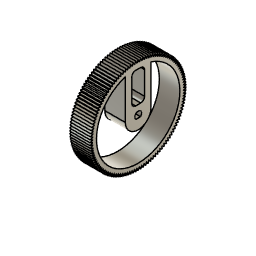
Whell Medium (Autodesk Fusion 360 design; units mm, degrees)
Autodesk Fusion 360 part; units mm, degrees
sketch "Sketch1" plane through (34, 0, 0) normal (-1, 0, 0) x (0, -1, 0)
  arc A0 (1.8888, -2) -> (-1.7388, -2) centre (0.075, 0) ccw
  line L0 (1.8888, -2) -> (-1.7388, -2)
  arc A1 (41.9734, -20.1687) -> (37.4682, -13) centre (37.4682, -18) ccw
  arc A2 (41.9734, 20.1687) -> (41.9734, -20.1687) centre (0.075, 0) ccw
  arc A3 (37.4682, 13) -> (41.9734, 20.1687) centre (37.4682, 18) ccw
  arc A4 (43.369, 3) -> (36.369, 10) centre (36.369, 3) ccw
  line L1 (43.369, 3) -> (43.369, -2.9712)
  arc A5 (36.369, -9.9712) -> (43.369, -2.9712) centre (36.369, -2.9712) ccw
  arc A6 (14.223, -2.9712) -> (21.223, -9.9712) centre (21.223, -2.9712) ccw
  line L2 (14.223, -2.9712) -> (14.223, 3)
  arc A7 (21.223, 10) -> (14.223, 3) centre (21.223, 3) ccw
  arc A8 (50.075, -0.0217) -> (50.075, 0.0217) centre (0.075, 0) ccw
  line L3 (50.075, 0.0217) -> (51.2929, 5.3832)
  line L4 (51.2929, 5.3832) -> (48.9869, 10.3743)
  arc A9 (48.9869, 10.3743) -> (48.9779, 10.4168) centre (0.075, 0) ccw
  line L5 (48.9779, 10.4168) -> (49.0544, 15.9144)
  line L6 (49.0544, 15.9144) -> (45.7611, 20.317)
  arc A10 (45.7611, 20.317) -> (45.7434, 20.3567) centre (0.075, 0) ccw
  line L7 (45.7434, 20.3567) -> (44.6753, 25.75)
  line L8 (44.6753, 25.75) -> (40.5386, 29.3717)
  arc A11 (40.5386, 29.3717) -> (40.5131, 29.4068) centre (0.075, 0) ccw
  line L9 (40.5131, 29.4068) -> (38.347, 34.4602)
  line L10 (38.347, 34.4602) -> (33.5477, 37.1427)
  arc A12 (33.5477, 37.1427) -> (33.5154, 37.1718) centre (0.075, 0) ccw
  line L11 (33.5154, 37.1718) -> (30.3459, 41.6644)
  line L12 (30.3459, 41.6644) -> (25.0938, 43.2904)
  arc A13 (25.0938, 43.2904) -> (25.0562, 43.3121) centre (0.075, 0) ccw
  line L13 (25.0562, 43.3121) -> (21.0219, 47.0476)
  line L14 (21.0219, 47.0476) -> (15.5465, 47.5461)
  arc A14 (15.5465, 47.5461) -> (15.5052, 47.5595) centre (0.075, 0) ccw
  line L15 (15.5052, 47.5595) -> (10.7825, 50.3746)
  line L16 (10.7825, 50.3746) -> (5.323, 49.7238)
  arc A15 (5.323, 49.7238) -> (5.2798, 49.7284) centre (0.075, 0) ccw
  line L17 (5.2798, 49.7284) -> (0.075, 51.5)
  line L18 (0.075, 51.5) -> (-5.1298, 49.7284)
  arc A16 (-5.1298, 49.7284) -> (-5.173, 49.7238) centre (0.075, 0) ccw
  line L19 (-5.173, 49.7238) -> (-10.6325, 50.3746)
  line L20 (-10.6325, 50.3746) -> (-15.3552, 47.5595)
  arc A17 (-15.3552, 47.5595) -> (-15.3965, 47.5461) centre (0.075, 0) ccw
  line L21 (-15.3965, 47.5461) -> (-20.8719, 47.0476)
  line L22 (-20.8719, 47.0476) -> (-24.9062, 43.3121)
  arc A18 (-24.9062, 43.3121) -> (-24.9438, 43.2904) centre (0.075, 0) ccw
  line L23 (-24.9438, 43.2904) -> (-30.1959, 41.6644)
  line L24 (-30.1959, 41.6644) -> (-33.3654, 37.1718)
  arc A19 (-33.3654, 37.1718) -> (-33.3977, 37.1427) centre (0.075, 0) ccw
  line L25 (-33.3977, 37.1427) -> (-38.197, 34.4602)
  line L26 (-38.197, 34.4602) -> (-40.3631, 29.4068)
  arc A20 (-40.3631, 29.4068) -> (-40.3886, 29.3717) centre (0.075, 0) ccw
  line L27 (-40.3886, 29.3717) -> (-44.5253, 25.75)
  line L28 (-44.5253, 25.75) -> (-45.5934, 20.3567)
  arc A21 (-45.5934, 20.3567) -> (-45.6111, 20.317) centre (0.075, 0) ccw
  line L29 (-45.6111, 20.317) -> (-48.9044, 15.9144)
  line L30 (-48.9044, 15.9144) -> (-48.8279, 10.4168)
  arc A22 (-48.8279, 10.4168) -> (-48.8369, 10.3743) centre (0.075, 0) ccw
  line L31 (-48.8369, 10.3743) -> (-51.1429, 5.3832)
  line L32 (-51.1429, 5.3832) -> (-49.925, 0.0217)
  arc A23 (-49.925, 0.0217) -> (-49.925, -0.0217) centre (0.075, 0) ccw
  line L33 (-49.925, -0.0217) -> (-51.1429, -5.3832)
  line L34 (-51.1429, -5.3832) -> (-48.8369, -10.3743)
  arc A24 (-48.8369, -10.3743) -> (-48.8279, -10.4168) centre (0.075, 0) ccw
  line L35 (-48.8279, -10.4168) -> (-48.9044, -15.9144)
  line L36 (-48.9044, -15.9144) -> (-45.6111, -20.317)
  arc A25 (-45.6111, -20.317) -> (-45.5934, -20.3567) centre (0.075, 0) ccw
  line L37 (-45.5934, -20.3567) -> (-44.5253, -25.75)
  line L38 (-44.5253, -25.75) -> (-40.3886, -29.3717)
  arc A26 (-40.3886, -29.3717) -> (-40.3631, -29.4068) centre (0.075, 0) ccw
  line L39 (-40.3631, -29.4068) -> (-38.197, -34.4602)
  line L40 (-38.197, -34.4602) -> (-33.3977, -37.1427)
  arc A27 (-33.3977, -37.1427) -> (-33.3654, -37.1718) centre (0.075, 0) ccw
  line L41 (-33.3654, -37.1718) -> (-30.1959, -41.6644)
  line L42 (-30.1959, -41.6644) -> (-24.9438, -43.2904)
  arc A28 (-24.9438, -43.2904) -> (-24.9062, -43.3121) centre (0.075, 0) ccw
  line L43 (-24.9062, -43.3121) -> (-20.8719, -47.0476)
  line L44 (-20.8719, -47.0476) -> (-15.3965, -47.5461)
  arc A29 (-15.3965, -47.5461) -> (-15.3552, -47.5595) centre (0.075, 0) ccw
  line L45 (-15.3552, -47.5595) -> (-10.6325, -50.3746)
  line L46 (-10.6325, -50.3746) -> (-5.173, -49.7238)
  arc A30 (-5.173, -49.7238) -> (-5.1298, -49.7284) centre (0.075, 0) ccw
  line L47 (-5.1298, -49.7284) -> (0.075, -51.5)
  line L48 (0.075, -51.5) -> (5.2798, -49.7284)
  arc A31 (5.2798, -49.7284) -> (5.323, -49.7238) centre (0.075, 0) ccw
  line L49 (5.323, -49.7238) -> (10.7825, -50.3746)
  line L50 (10.7825, -50.3746) -> (15.5052, -47.5595)
  arc A32 (15.5052, -47.5595) -> (15.5465, -47.5461) centre (0.075, 0) ccw
  line L51 (15.5465, -47.5461) -> (21.0219, -47.0476)
  line L52 (21.0219, -47.0476) -> (25.0562, -43.3121)
  arc A33 (25.0562, -43.3121) -> (25.0938, -43.2904) centre (0.075, 0) ccw
  line L53 (25.0938, -43.2904) -> (30.3459, -41.6644)
  line L54 (30.3459, -41.6644) -> (33.5154, -37.1718)
  arc A34 (33.5154, -37.1718) -> (33.5477, -37.1427) centre (0.075, 0) ccw
  line L55 (33.5477, -37.1427) -> (38.347, -34.4602)
  line L56 (38.347, -34.4602) -> (40.5131, -29.4068)
  arc A35 (40.5131, -29.4068) -> (40.5386, -29.3717) centre (0.075, 0) ccw
  line L57 (40.5386, -29.3717) -> (44.6753, -25.75)
  line L58 (44.6753, -25.75) -> (45.7434, -20.3567)
  arc A36 (45.7434, -20.3567) -> (45.7611, -20.317) centre (0.075, 0) ccw
  line L59 (45.7611, -20.317) -> (49.0544, -15.9144)
  line L60 (49.0544, -15.9144) -> (48.9779, -10.4168)
  arc A37 (48.9779, -10.4168) -> (48.9869, -10.3743) centre (0.075, 0) ccw
  line L61 (48.9869, -10.3743) -> (51.2929, -5.3832)
  line L62 (51.2929, -5.3832) -> (50.075, -0.0217)
  arc A38 (1.8888, -2) -> (-1.7388, -2) centre (0.075, 0) ccw
  line L63 (1.8888, -2) -> (-1.7388, -2)
  circle A39 centre (0.075, 0) radius 37.5
  line L64 (0.075, 0) -> (0.075, 37.5) construction
  line L65 (0.075, 37.5) -> (-1.0186, 34.9829)
  line L66 (0.075, 37.5) -> (1.1677, 34.9829)
  line L67 (-1.8876, 37.4486) -> (-0.6647, 34.9922)
  line L68 (-1.8876, 37.4486) -> (-2.8479, 34.8777)
  line L69 (-3.8448, 37.2946) -> (-2.495, 34.9055)
  line L70 (-3.8448, 37.2946) -> (-4.6693, 34.677)
  line L71 (-5.7913, 37.0383) -> (-4.3183, 34.7232)
  line L72 (-5.7913, 37.0383) -> (-6.4776, 34.3811)
  line L73 (-7.7217, 36.6805) -> (-6.1296, 34.4457)
  line L74 (-7.7217, 36.6805) -> (-8.268, 33.9911)
  line L75 (-9.6307, 36.2222) -> (-7.9238, 34.0737)
  line L76 (-9.6307, 36.2222) -> (-10.0355, 33.5079)
  line L77 (-11.5131, 35.6646) -> (-9.6961, 33.6084)
  line L78 (-11.5131, 35.6646) -> (-11.7754, 32.9328)
  line L79 (-13.3638, 35.0093) -> (-11.4417, 33.051)
  line L80 (-13.3638, 35.0093) -> (-13.4827, 32.2675)
  line L81 (-15.1776, 34.258) -> (-13.1556, 32.4029)
  line L82 (-15.1776, 34.258) -> (-15.1529, 31.5137)
  line L83 (-16.9496, 33.4127) -> (-14.8333, 31.6661)
  line L84 (-16.9496, 33.4127) -> (-16.7813, 30.6735)
  line L85 (-18.675, 32.476) -> (-16.4702, 30.8425)
  line L86 (-18.675, 32.476) -> (-18.3635, 29.7493)
  line L87 (-20.349, 31.4501) -> (-18.0617, 29.9343)
  line L88 (-20.349, 31.4501) -> (-19.8952, 28.7435)
  line L89 (-21.9669, 30.3381) -> (-19.6035, 28.9441)
  line L90 (-21.9669, 30.3381) -> (-21.3722, 27.659)
  line L91 (-23.5245, 29.143) -> (-21.0913, 27.8745)
  line L92 (-23.5245, 29.143) -> (-22.7903, 26.4986)
  line L93 (-25.0174, 27.8679) -> (-22.5211, 26.7285)
  line L94 (-25.0174, 27.8679) -> (-24.1458, 25.2656)
  line L95 (-26.4415, 26.5165) -> (-23.889, 25.5093)
  line L96 (-26.4415, 26.5165) -> (-25.4349, 23.9634)
  line L97 (-27.7929, 25.0924) -> (-25.1912, 24.2202)
  line L98 (-27.7929, 25.0924) -> (-26.6541, 22.5955)
  line L99 (-29.068, 23.5995) -> (-26.4242, 22.8646)
  line L100 (-29.068, 23.5995) -> (-27.8, 21.1656)
  line L101 (-30.2631, 22.0419) -> (-27.5845, 21.4465)
  line L102 (-30.2631, 22.0419) -> (-28.8696, 19.6777)
  line L103 (-31.3751, 20.424) -> (-28.669, 19.9695)
  line L104 (-31.3751, 20.424) -> (-29.8597, 18.1359)
  line L105 (-32.401, 18.75) -> (-29.6748, 18.4378)
  line L106 (-32.401, 18.75) -> (-30.7679, 16.5444)
  line L107 (-33.3377, 17.0246) -> (-30.599, 16.8555)
  line L108 (-33.3377, 17.0246) -> (-31.5915, 14.9075)
  line L109 (-34.183, 15.2526) -> (-31.4391, 15.2271)
  line L110 (-34.183, 15.2526) -> (-32.3283, 13.2298)
  line L111 (-34.9343, 13.4388) -> (-32.1928, 13.5569)
  line L112 (-34.9343, 13.4388) -> (-32.9763, 11.5158)
  line L113 (-35.5896, 11.5881) -> (-32.8581, 11.8495)
  line L114 (-35.5896, 11.5881) -> (-33.5337, 9.7703)
  line L115 (-36.1472, 9.7057) -> (-33.4331, 10.1097)
  line L116 (-36.1472, 9.7057) -> (-33.9989, 7.9979)
  line L117 (-36.6055, 7.7967) -> (-33.9163, 8.3422)
  line L118 (-36.6055, 7.7967) -> (-34.3708, 6.2037)
  line L119 (-36.9633, 5.8663) -> (-34.3063, 6.5518)
  line L120 (-36.9633, 5.8663) -> (-34.6483, 4.3924)
  line L121 (-37.2196, 3.9198) -> (-34.6021, 4.7434)
  line L122 (-37.2196, 3.9198) -> (-34.8306, 2.5691)
  line L123 (-37.3736, 1.9626) -> (-34.8028, 2.922)
  line L124 (-37.3736, 1.9626) -> (-34.9172, 0.7388)
  line L125 (-37.425, 0) -> (-34.9079, 1.0927)
  line L126 (-37.425, 0) -> (-34.9079, -1.0936)
  line L127 (-37.3736, -1.9626) -> (-34.9172, -0.7397)
  line L128 (-37.3736, -1.9626) -> (-34.8027, -2.9229)
  line L129 (-37.2196, -3.9198) -> (-34.8305, -2.57)
  line L130 (-37.2196, -3.9198) -> (-34.602, -4.7443)
  line L131 (-36.9633, -5.8663) -> (-34.6482, -4.3933)
  line L132 (-36.9633, -5.8663) -> (-34.3061, -6.5526)
  line L133 (-36.6055, -7.7967) -> (-34.3707, -6.2046)
  line L134 (-36.6055, -7.7967) -> (-33.9161, -8.343)
  line L135 (-36.1472, -9.7057) -> (-33.9987, -7.9988)
  line L136 (-36.1472, -9.7057) -> (-33.4329, -10.1105)
  line L137 (-35.5896, -11.5881) -> (-33.5334, -9.7711)
  line L138 (-35.5896, -11.5881) -> (-32.8578, -11.8504)
  line L139 (-34.9343, -13.4388) -> (-32.976, -11.5167)
  line L140 (-34.9343, -13.4388) -> (-32.1925, -13.5577)
  line L141 (-34.183, -15.2526) -> (-32.3279, -13.2306)
  line L142 (-34.183, -15.2526) -> (-31.4387, -15.2279)
  line L143 (-33.3377, -17.0246) -> (-31.5911, -14.9083)
  line L144 (-33.3377, -17.0246) -> (-30.5985, -16.8563)
  line L145 (-32.401, -18.75) -> (-30.7675, -16.5452)
  line L146 (-32.401, -18.75) -> (-29.6743, -18.4385)
  line L147 (-31.3751, -20.424) -> (-29.8593, -18.1367)
  line L148 (-31.3751, -20.424) -> (-28.6685, -19.9702)
  line L149 (-30.2631, -22.0419) -> (-28.8691, -19.6785)
  line L150 (-30.2631, -22.0419) -> (-27.584, -21.4472)
  line L151 (-29.068, -23.5995) -> (-27.7995, -21.1663)
  line L152 (-29.068, -23.5995) -> (-26.4236, -22.8653)
  line L153 (-27.7929, -25.0924) -> (-26.6535, -22.5961)
  line L154 (-27.7929, -25.0924) -> (-25.1906, -24.2208)
  line L155 (-26.4415, -26.5165) -> (-25.4343, -23.964)
  line L156 (-26.4415, -26.5165) -> (-23.8884, -25.5099)
  line L157 (-25.0174, -27.8679) -> (-24.1452, -25.2662)
  line L158 (-25.0174, -27.8679) -> (-22.5205, -26.7291)
  line L159 (-23.5245, -29.143) -> (-22.7896, -26.4992)
  line L160 (-23.5245, -29.143) -> (-21.0906, -27.875)
  line L161 (-21.9669, -30.3381) -> (-21.3715, -27.6595)
  line L162 (-21.9669, -30.3381) -> (-19.6027, -28.9446)
  line L163 (-20.349, -31.4501) -> (-19.8945, -28.744)
  line L164 (-20.349, -31.4501) -> (-18.0609, -29.9347)
  line L165 (-18.675, -32.476) -> (-18.3628, -29.7498)
  line L166 (-18.675, -32.476) -> (-16.4694, -30.8429)
  line L167 (-16.9496, -33.4127) -> (-16.7805, -30.674)
  line L168 (-16.9496, -33.4127) -> (-14.8325, -31.6665)
  line L169 (-15.1776, -34.258) -> (-15.1521, -31.5141)
  line L170 (-15.1776, -34.258) -> (-13.1548, -32.4033)
  line L171 (-13.3638, -35.0093) -> (-13.4819, -32.2678)
  line L172 (-13.3638, -35.0093) -> (-11.4408, -33.0513)
  line L173 (-11.5131, -35.6646) -> (-11.7745, -32.9331)
  line L174 (-11.5131, -35.6646) -> (-9.6953, -33.6087)
  line L175 (-9.6307, -36.2222) -> (-10.0347, -33.5081)
  line L176 (-9.6307, -36.2222) -> (-7.9229, -34.0739)
  line L177 (-7.7217, -36.6805) -> (-8.2672, -33.9913)
  line L178 (-7.7217, -36.6805) -> (-6.1287, -34.4458)
  line L179 (-5.7913, -37.0383) -> (-6.4768, -34.3813)
  line L180 (-5.7913, -37.0383) -> (-4.3174, -34.7233)
  line L181 (-3.8448, -37.2946) -> (-4.6684, -34.6771)
  line L182 (-3.8448, -37.2946) -> (-2.4941, -34.9056)
  line L183 (-1.8876, -37.4486) -> (-2.847, -34.8778)
  line L184 (-1.8876, -37.4486) -> (-0.6638, -34.9922)
  line L185 (0.075, -37.5) -> (-1.0177, -34.9829)
  line L186 (0.075, -37.5) -> (1.1686, -34.9829)
  line L187 (2.0376, -37.4486) -> (0.8147, -34.9922)
  line L188 (2.0376, -37.4486) -> (2.9979, -34.8777)
  line L189 (3.9948, -37.2946) -> (2.645, -34.9055)
  line L190 (3.9948, -37.2946) -> (4.8193, -34.677)
  line L191 (5.9413, -37.0383) -> (4.4683, -34.7232)
  line L192 (5.9413, -37.0383) -> (6.6276, -34.3811)
  line L193 (7.8717, -36.6805) -> (6.2796, -34.4457)
  line L194 (7.8717, -36.6805) -> (8.418, -33.9911)
  line L195 (9.7807, -36.2222) -> (8.0738, -34.0737)
  line L196 (9.7807, -36.2222) -> (10.1855, -33.5079)
  line L197 (11.6631, -35.6646) -> (9.8461, -33.6084)
  line L198 (11.6631, -35.6646) -> (11.9254, -32.9328)
  line L199 (13.5138, -35.0093) -> (11.5917, -33.051)
  line L200 (13.5138, -35.0093) -> (13.6327, -32.2675)
  line L201 (15.3276, -34.258) -> (13.3056, -32.4029)
  line L202 (15.3276, -34.258) -> (15.3029, -31.5137)
  line L203 (17.0996, -33.4127) -> (14.9833, -31.6661)
  line L204 (17.0996, -33.4127) -> (16.9313, -30.6735)
  line L205 (18.825, -32.476) -> (16.6202, -30.8425)
  line L206 (18.825, -32.476) -> (18.5135, -29.7493)
  line L207 (20.499, -31.4501) -> (18.2117, -29.9343)
  line L208 (20.499, -31.4501) -> (20.0452, -28.7435)
  line L209 (22.1169, -30.3381) -> (19.7535, -28.9441)
  line L210 (22.1169, -30.3381) -> (21.5222, -27.659)
  line L211 (23.6745, -29.143) -> (21.2413, -27.8745)
  line L212 (23.6745, -29.143) -> (22.9403, -26.4986)
  line L213 (25.1674, -27.8679) -> (22.6711, -26.7285)
  line L214 (25.1674, -27.8679) -> (24.2958, -25.2656)
  line L215 (26.5915, -26.5165) -> (24.039, -25.5093)
  line L216 (26.5915, -26.5165) -> (25.5849, -23.9634)
  line L217 (27.9429, -25.0924) -> (25.3412, -24.2202)
  line L218 (27.9429, -25.0924) -> (26.8041, -22.5955)
  line L219 (29.218, -23.5995) -> (26.5742, -22.8646)
  line L220 (29.218, -23.5995) -> (27.95, -21.1656)
  line L221 (30.4131, -22.0419) -> (27.7345, -21.4465)
  line L222 (30.4131, -22.0419) -> (29.0195, -19.6777)
  line L223 (31.5251, -20.424) -> (28.819, -19.9695)
  line L224 (31.5251, -20.424) -> (30.0097, -18.1359)
  line L225 (32.551, -18.75) -> (29.8248, -18.4378)
  line L226 (32.551, -18.75) -> (30.9179, -16.5444)
  line L227 (33.4877, -17.0246) -> (30.749, -16.8555)
  line L228 (33.4877, -17.0246) -> (31.7415, -14.9075)
  line L229 (34.333, -15.2526) -> (31.5891, -15.2271)
  line L230 (34.333, -15.2526) -> (32.4783, -13.2298)
  line L231 (35.0843, -13.4388) -> (32.3428, -13.5569)
  line L232 (35.0843, -13.4388) -> (33.1263, -11.5158)
  line L233 (35.7396, -11.5881) -> (33.0081, -11.8495)
  line L234 (35.7396, -11.5881) -> (33.6837, -9.7703)
  line L235 (36.2972, -9.7057) -> (33.5831, -10.1097)
  line L236 (36.2972, -9.7057) -> (34.1489, -7.9979)
  line L237 (36.7555, -7.7967) -> (34.0663, -8.3422)
  line L238 (36.7555, -7.7967) -> (34.5208, -6.2037)
  line L239 (37.1133, -5.8663) -> (34.4563, -6.5518)
  line L240 (37.1133, -5.8663) -> (34.7983, -4.3924)
  line L241 (37.3696, -3.9198) -> (34.7521, -4.7434)
  line L242 (37.3696, -3.9198) -> (34.9806, -2.5691)
  line L243 (37.5236, -1.9626) -> (34.9528, -2.922)
  line L244 (37.5236, -1.9626) -> (35.0672, -0.7388)
  line L245 (37.575, 0) -> (35.0579, -1.0927)
  line L246 (37.575, 0) -> (35.0579, 1.0936)
  line L247 (37.5236, 1.9626) -> (35.0672, 0.7397)
  line L248 (37.5236, 1.9626) -> (34.9527, 2.9229)
  line L249 (37.3696, 3.9198) -> (34.9805, 2.57)
  line L250 (37.3696, 3.9198) -> (34.752, 4.7443)
  line L251 (37.1133, 5.8663) -> (34.7982, 4.3933)
  line L252 (37.1133, 5.8663) -> (34.4561, 6.5526)
  line L253 (36.7555, 7.7967) -> (34.5207, 6.2046)
  line L254 (36.7555, 7.7967) -> (34.0661, 8.343)
  line L255 (36.2972, 9.7057) -> (34.1487, 7.9988)
  line L256 (36.2972, 9.7057) -> (33.5829, 10.1105)
  line L257 (35.7396, 11.5881) -> (33.6834, 9.7711)
  line L258 (35.7396, 11.5881) -> (33.0078, 11.8504)
  line L259 (35.0843, 13.4388) -> (33.126, 11.5167)
  line L260 (35.0843, 13.4388) -> (32.3425, 13.5577)
  line L261 (34.333, 15.2526) -> (32.4779, 13.2306)
  line L262 (34.333, 15.2526) -> (31.5887, 15.2279)
  line L263 (33.4877, 17.0246) -> (31.7411, 14.9083)
  line L264 (33.4877, 17.0246) -> (30.7485, 16.8563)
  line L265 (32.551, 18.75) -> (30.9175, 16.5452)
  line L266 (32.551, 18.75) -> (29.8243, 18.4385)
  line L267 (31.5251, 20.424) -> (30.0093, 18.1367)
  line L268 (31.5251, 20.424) -> (28.8185, 19.9702)
  line L269 (30.4131, 22.0419) -> (29.0191, 19.6785)
  line L270 (30.4131, 22.0419) -> (27.734, 21.4472)
  line L271 (29.218, 23.5995) -> (27.9495, 21.1663)
  line L272 (29.218, 23.5995) -> (26.5736, 22.8653)
  line L273 (27.9429, 25.0924) -> (26.8035, 22.5961)
  line L274 (27.9429, 25.0924) -> (25.3406, 24.2208)
  line L275 (26.5915, 26.5165) -> (25.5843, 23.964)
  line L276 (26.5915, 26.5165) -> (24.0384, 25.5099)
  line L277 (25.1674, 27.8679) -> (24.2952, 25.2662)
  line L278 (25.1674, 27.8679) -> (22.6705, 26.7291)
  line L279 (23.6745, 29.143) -> (22.9396, 26.4992)
  line L280 (23.6745, 29.143) -> (21.2406, 27.875)
  line L281 (22.1169, 30.3381) -> (21.5215, 27.6595)
  line L282 (22.1169, 30.3381) -> (19.7527, 28.9446)
  line L283 (20.499, 31.4501) -> (20.0445, 28.744)
  line L284 (20.499, 31.4501) -> (18.2109, 29.9347)
  line L285 (18.825, 32.476) -> (18.5128, 29.7498)
  line L286 (18.825, 32.476) -> (16.6194, 30.8429)
  line L287 (17.0996, 33.4127) -> (16.9305, 30.674)
  line L288 (17.0996, 33.4127) -> (14.9825, 31.6665)
  line L289 (15.3276, 34.258) -> (15.3021, 31.5141)
  line L290 (15.3276, 34.258) -> (13.3048, 32.4033)
  line L291 (13.5138, 35.0093) -> (13.6319, 32.2678)
  line L292 (13.5138, 35.0093) -> (11.5908, 33.0513)
  line L293 (11.6631, 35.6646) -> (11.9245, 32.9331)
  line L294 (11.6631, 35.6646) -> (9.8453, 33.6087)
  line L295 (9.7807, 36.2222) -> (10.1847, 33.5081)
  line L296 (9.7807, 36.2222) -> (8.0729, 34.0739)
  line L297 (7.8717, 36.6805) -> (8.4172, 33.9913)
  line L298 (7.8717, 36.6805) -> (6.2787, 34.4458)
  line L299 (5.9413, 37.0383) -> (6.6268, 34.3813)
  line L300 (5.9413, 37.0383) -> (4.4674, 34.7233)
  line L301 (3.9948, 37.2946) -> (4.8184, 34.6771)
  line L302 (3.9948, 37.2946) -> (2.6441, 34.9056)
  line L303 (2.0376, 37.4486) -> (2.997, 34.8778)
  line L304 (2.0376, 37.4486) -> (0.8138, 34.9922)
  line L305 (-9.925, 0) -> (-9.925, 30.9233)
  line L306 (10.075, 0) -> (10.075, 30.9233)
  arc A40 (-9.925, 0) -> (10.075, 0) centre (0.075, 0) ccw
  arc A41 (-9.925, 30.9233) -> (10.075, 30.9233) centre (0.075, 0) ccw
  line L307 (2.075, 7.1628) -> (-1.925, 7.1628)
  line L308 (-4.925, 10.1628) -> (-4.925, 28.1628)
  line L309 (-1.925, 31.1628) -> (2.075, 31.1628)
  line L310 (5.075, 28.1628) -> (5.075, 10.1628)
  line L311 (5.075, 7.1628) -> (-4.925, 31.1628) construction
  line L312 (-4.925, 7.1628) -> (5.075, 31.1628) construction
  arc A42 (-4.925, 10.1628) -> (-1.925, 7.1628) centre (-1.925, 10.1628) ccw
  arc A43 (2.075, 7.1628) -> (5.075, 10.1628) centre (2.075, 10.1628) ccw
  arc A44 (5.075, 28.1628) -> (2.075, 31.1628) centre (2.075, 28.1628) ccw
  arc A45 (-1.925, 31.1628) -> (-4.925, 28.1628) centre (-1.925, 28.1628) ccw
  point P0 (0.075, 19.1628)
  dimension "d375" = 75
  dimension "d376" = 2.744
  dimension "d378" = 360
  dimension "d379" = 65
  dimension "d381" = 10
  dimension "d382" = 24
  dimension "d383" = 3
  constraint concentric A37 A39
  constraint coincident A0.centre A2.centre
  constraint coincident A39 L64.end
  constraint vertical L64
  constraint concentric A36 A41
  constraint concentric A36 A40
  constraint tangent L305 A40
  constraint tangent L306 A40
  constraint horizontal L307
  constraint perpendicular L307 L308
  constraint parallel L307 L309
  constraint parallel L308 L310
  constraint coincident L311 P0
  constraint coincident L312 P0
  constraint coincident L64 P0
  constraint coincident L312.start L307
  constraint coincident L312.start L308
  constraint tangent L307 A42
  constraint tangent L308 A42
  constraint coincident L311.start L307
  constraint coincident L311.start L310
  constraint tangent L307 A43
  constraint tangent L310 A43
  constraint equal A42 A43
  constraint coincident L312.end L309
  constraint coincident L312.end L310
  constraint tangent L309 A44
  constraint tangent L310 A44
  constraint equal A42 A44
  constraint coincident L311.end L308
  constraint coincident L311.end L309
  constraint tangent L308 A45
  constraint tangent L309 A45
  constraint equal A42 A45
  measures "d375" diameter of A39
  measures "d376" distance of L64.end L66.end
  measures "d379" diameter of A41
  measures "d381" distance of L311.end L312.end
  measures "d382" distance of L312.start L311.end
  measures "d383" radius of A42
extrude "Extrude1" add sketch "Sketch1" against normal blind 16 contours L65 L66 L67 L68 L69 L70 L71 L72 L73 L74 L75 L76 L77 L78 L79 L80 L81 L82 L83 L84 L85 L86 L87 L88 L89 L90 L91 L92 L93 L94 L95 L96 L97 L98 L99 L100 L101 L102 L103 L104 L105 L106 L107 L108 L109 L110 L111 L112 L113 L114 L115 L116 L117 L118 L119 L120 L121 L122 L123 L124 L125 L126 L127 L128 L129 L130 L131 L132 L133 L134 L135 L136 L137 L138 L139 L140 L141 L142 L143 L144 L145 L146 L147 L148 L149 L150 L151 L152 L153 L154 L155 L156 L157 L158 L159 L160 L161 L162 L163 L164 L165 L166 L167 L168 L169 L170 L171 L172 L173 L174 L175 L176 L177 L178 L179 L180 L181 L182 L183 L184 L185 L186 L187 L188 L189 L190 L191 L192 L193 L194 L195 L196 L197 L198 L199 L200 L201 L202 L203 L204 L205 L206 L207 L208 L209 L210 L211 L212 L213 L214 L215 L216 L217 L218 L219 L220 L221 L222 L223 L224 L225 L226 L227 L228 L229 L230 L231 L232 L233 L234 L235 L236 L237 L238 L239 L240 L241 L242 L243 L244 L245 L246 L247 L248 L249 L250 L251 L252 L253 L254 L255 L256 L257 L258 L259 L260 L261 L262 L263 L264 L265 L266 L267 L268 L269 L270 L271 L272 L273 L274 L275 L276 L277 L278 L279 L280 L281 L282 L283 L284 L285 L286 L287 L288 L289 L290 L291 L292 L293 L294 L295 L296 L297 L298 L299 L300 L301 L302 L303 L304
